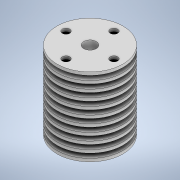
# Autodesk Inventor part: Radiator
Saved by Autodesk Inventor 2022 (Build 260153000, 153)
## iProperties
Created: 2023-12-26
Part Number: Radiator
Material: Типовые
Document SubType Name: Modeling
Designer: Admin
Density: 1 g/cm^3
Appearance: По умолчанию
Author: Admin
Autodesk Inventor part; units mm, degrees
ref_plane "YZ Plane" through (0, 0, 0) normal (1, 0, 0) x (0, 1, 0)
ref_plane "XZ Plane" through (0, 0, 0) normal (0, 1, 0) x (-1, 0, 0)
ref_plane "XY Plane" through (0, 0, 0) normal (0, 0, 1) x (1, 0, 0)
sketch "Эскиз1" plane through (0, 0, 0) normal (0, 0, 1) x (1, 0, 0)
  line L0 (11, 0.5) -> (-11, 0.5)
  line L1 (-11, 0.5) -> (-11, -0.5)
  line L2 (-11, -0.5) -> (11, -0.5)
  line L3 (11, -0.5) -> (11, 0.5)
  line L4 (11, 0.5) -> (-11, -0.5) construction
  line L5 (-11, 0.5) -> (11, -0.5) construction
  line L6 (-11, 2) -> (11, 2)
  line L7 (11, 2) -> (11, 3)
  line L8 (11, 3) -> (-11, 3)
  line L9 (-11, 3) -> (-11, 2)
  line L10 (-11, 4.5) -> (11, 4.5)
  line L11 (11, 4.5) -> (11, 5.5)
  line L12 (11, 5.5) -> (-11, 5.5)
  line L13 (-11, 5.5) -> (-11, 4.5)
  line L14 (-11, 7) -> (11, 7)
  line L15 (11, 7) -> (11, 8)
  line L16 (11, 8) -> (-11, 8)
  line L17 (-11, 8) -> (-11, 7)
  line L18 (-11, 9.5) -> (11, 9.5)
  line L19 (11, 9.5) -> (11, 10.5)
  line L20 (11, 10.5) -> (-11, 10.5)
  line L21 (-11, 10.5) -> (-11, 9.5)
  line L22 (-11, 12) -> (11, 12)
  line L23 (11, 12) -> (11, 13)
  line L24 (11, 13) -> (-11, 13)
  line L25 (-11, 13) -> (-11, 12)
  line L26 (-11, 14.5) -> (11, 14.5)
  line L27 (11, 14.5) -> (11, 15.5)
  line L28 (11, 15.5) -> (-11, 15.5)
  line L29 (-11, 15.5) -> (-11, 14.5)
  line L30 (-11, 17) -> (11, 17)
  line L31 (11, 17) -> (11, 18)
  line L32 (11, 18) -> (-11, 18)
  line L33 (-11, 18) -> (-11, 17)
  line L34 (-11, 19.5) -> (11, 19.5)
  line L35 (11, 19.5) -> (11, 20.5)
  line L36 (11, 20.5) -> (-11, 20.5)
  line L37 (-11, 20.5) -> (-11, 19.5)
  line L38 (-11, 22) -> (11, 22)
  line L39 (11, 22) -> (11, 23)
  line L40 (11, 23) -> (-11, 23)
  line L41 (-11, 23) -> (-11, 22)
  line L42 (-11, 24.5) -> (11, 24.5)
  line L43 (11, 24.5) -> (11, 25.5)
  line L44 (11, 25.5) -> (-11, 25.5)
  line L45 (-11, 25.5) -> (-11, 24.5)
  line L46 (0, -0.5) -> (0, 25.5)
  circle A0 centre (0, 24.5) radius 4.8 construction
  circle A1 centre (0, 0.5) radius 6 construction
  line L47 (-6, 0.5) -> (-4.8, 24.5)
  line L48 (6, 0.5) -> (4.8, 24.5)
  point P0 (0, 0)
  point P1 (0, 0)
  point P2 (0, 2)
  point P3 (0, 3)
  point P4 (0, 4.5)
  point P5 (0, 7)
  point P6 (0, 5.5)
  point P7 (0, 9.5)
  point P8 (0, 8)
  point P9 (0, 12)
  point P10 (0, 10.5)
  point P11 (0, 14.5)
  point P12 (0, 13)
  point P13 (0, 17)
  point P14 (0, 15.5)
  point P15 (0, 18)
  point P16 (0, 19.5)
  point P17 (0, 22)
  point P18 (0, 20.5)
  point P19 (-4.925, 22)
  point P20 (-4.875, 23)
  point P21 (-5.125, 18)
  point P22 (-5.175, 17)
  point P23 (-5.25, 15.5)
  point P24 (-5.3, 14.5)
  point P25 (-5.375, 13)
  point P26 (-5.425, 12)
  point P27 (-5.5, 10.5)
  point P28 (0, 9.5)
  point P29 (0, 22)
  point P30 (0, 23)
  point P31 (-5.675, 7)
  point P32 (-5.625, 8)
  point P33 (-5.8, 4.5)
  point P34 (-5.75, 5.5)
  point P35 (-5.875, 3)
  point P36 (-5.925, 2)
  point P37 (0, 4.5)
  point P38 (0, 5.5)
  point P39 (0, 7)
  point P40 (-5.55, 9.5)
  point P41 (0, 8)
  point P42 (-5.05, 19.5)
  point P43 (-5, 20.5)
  dimension "d0" = 22
  dimension "d1" = 1
  dimension "d2" = 1.5
  dimension "d3" = 1.5
  dimension "d4" = 1.5
  dimension "d5" = 1.5
  dimension "d6" = 1.5
  dimension "d7" = 1.5
  dimension "d8" = 1.5
  dimension "d9" = 1.5
  dimension "d10" = 1.5
  dimension "d11" = 1
  dimension "d12" = 1
  dimension "d13" = 1
  dimension "d14" = 1
  dimension "d15" = 1
  dimension "d16" = 1
  dimension "d17" = 1
  dimension "d18" = 1
  dimension "d19" = 1
  dimension "d20" = 1
  dimension "d21" = 1.5
  dimension "d22" = 9.6
  dimension "d23" = 12
  constraints: 98 end point, 24 midpoint, 22 parallel, 16 vertical alignment, 11 horizontal, 11 perpendicular, 11 point on line, 4 point on circle, 2 centre point
  measures "d0" distance of L2.end L1.end
  measures "d1" distance of L1.end L0.end
  measures "d2" distance between parallel lines of L0 L6
  measures "d3" distance between parallel lines of L10 L8
  measures "d4" distance between parallel lines of L14 L12
  measures "d5" distance between parallel lines of L18 L16
  measures "d6" distance between parallel lines of L22 L20
  measures "d7" distance between parallel lines of L24 L26
  measures "d8" distance between parallel lines of L30 L28
  measures "d9" distance between parallel lines of L34 L32
  measures "d10" distance between parallel lines of L38 L36
  measures "d11" distance of L38.end L39.end
  measures "d12" distance of L34.end L35.end
  measures "d13" distance of L30.end L31.end
  measures "d14" distance of L26.end L27.end
  measures "d15" distance of L22.end L23.end
  measures "d16" distance of L18.end L19.end
  measures "d17" distance of L14.end L15.end
  measures "d18" distance of L10.end L11.end
  measures "d19" distance of L6.end L7.end
  measures "d20" distance of L44.end L42.start
  measures "d21" distance between parallel lines of L40 L42
  measures "d22" diameter of A0
  measures "d23" diameter of A1
revolve "Вращение1" add sketch "Эскиз1" angle 360 about axis through (0, -0.5, 0) along (0, 1, 0) contours L46 L2 L1 L0 | L0 L47 L6 L46 | L6 L47 L8 L46 | L6 L9 L8 L47 | L8 L47 L10 L46 | L10 L47 L12 L46 | L10 L13 L12 L47 | L12 L47 L14 L46 | L14 L47 L16 L46 | L14 L17 L16 L47 | L16 L47 L18 L46 | L18 L47 L20 L46 | L18 L21 L20 L47 | L20 L47 L22 L46 | L22 L47 L24 L46 | L22 L25 L24 L47 | L24 L47 L26 L46 | L26 L47 L28 L46 | L26 L29 L28 L47 | L28 L47 L30 L46 | L30 L47 L32 L46 | L30 L33 L32 L47 | L32 L47 L34 L46 | L34 L47 L36 L46 | L34 L37 L36 L47 | L36 L47 L38 L46 | L38 L47 L40 L46 | L38 L41 L40 L47 | L40 L47 L42 L46 | L42 L45 L44 L46
sketch "Эскиз2" plane through (0, -0.5, 0) normal (0, -1, 0) x (1, 0, 0)
  circle A0 centre (0, 0) radius 3.5
  dimension "d25" = 7
  constraints: 1 centre point, 1 coincident
  measures "d25" diameter of A0
extrude "Выдавливание1" cut sketch "Эскиз2" against normal blind 12
sketch "Эскиз3" plane through (0, 25.5, 0) normal (0, 1, 0) x (1, 0, 0)
  circle A0 centre (0, 0) radius 2.1
  dimension "d28" = 4.2
  constraints: 1 centre point, 1 coincident
  measures "d28" diameter of A0
extrude "Выдавливание2" cut sketch "Эскиз3" against normal through all
sketch "Эскиз4" plane through (0, 25.5, 0) normal (0, 1, 0) x (1, 0, 0)
  circle A0 centre (0, 0) radius 8 construction
  circle A1 centre (0, 8) radius 1.25
  circle A2 centre (-8, 0) radius 1.25
  circle A3 centre (0, -8) radius 1.25
  circle A4 centre (8, 0) radius 1.25
  dimension "d31" = 16
  dimension "d32" = 2.5
  dimension "d35" = 360
  constraints: 4 centre point, 2 vertical alignment, 1 coincident, 11 other
  measures "d32" diameter of A1
extrude "Выдавливание3" cut sketch "Эскиз4" against normal up to surface (3.5 mm away)
chamfer "Фаска1" distance 0.5 angle 45 1 edges at (-3.5, -0.5, 0)
